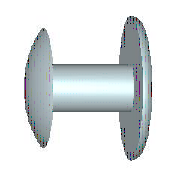
# Autodesk Inventor part: Rivet GB/T 1014-1986-2 X 4
Saved by Autodesk Inventor 2019 (Build 230136000, 136)
## iProperties
IsCustomPart: 0
Company: Autodesk Inc.
Created: 2017-02-09
Part Number: Rivet GB/T 1014-1986-2 X 4
Material: Steel, Mild
Description: Truss head semi - tubuar rivets
Document SubType Name: Modeling
Standard: GB/T 1014-1986
Designer: Autodesk Inc.
Standards Organization: GB
Language: en-US
Size Designation: 2-4
Categories: <MemberInstance><Categories><Category DisplayName="Fasteners" InternalName="e4da775c-781d-43d5-af7c-5136215cf5a6" Mnemonic="FSTN"><Category DisplayName="Rivets" InternalName="cf3d8c00-4198-4f00-854b-0d52b0adb238" Mnemonic="RIVET"><CategoryParameter DisplayName="Nominal Diameter" InternalName="0b221833-a430-4b2f-a4d4-a4e7cdbab5fe" Mnemonic="nomdia"/><CategoryParameter DisplayName="Nominal Length" InternalName="184b63f4-60b5-4ddb-b59d-a876aedee7db" Mnemonic="nomlen"/><CategoryParameter DisplayName="Functional Length" InternalName="2e4ddd0b-69f7-4d63-b45a-ef59153ff940" Mnemonic="fnclen"/><CategoryParameter DisplayName="Type" InternalName="841ce55c-7089-4646-bdbb-4888c77f269c" Mnemonic="type"/><CategoryParameter DisplayName="Grip Range (Min.-Max.)" InternalName="b095e0a4-6026-43f1-9b5f-1a93f7499cb0" Mnemonic="grprng"/></Category></Category><Category DisplayName="DataType" InternalName="23b78d0f-2648-40c6-8793-ca6db495c9e8" Mnemonic="DATATYPE"><CategoryParameter DisplayName="DisplayName" InternalName="05415f3d-3907-474b-a020-eb9d644f4cf3" Mnemonic="DISPLAYNAME"/><CategoryParameter DisplayName="Standard" InternalName="0c0a119c-1e12-4c84-803f-101930972f5e" Mnemonic="STANDARD"/><CategoryParameter DisplayName="Description" InternalName="13903e3d-64b1-4950-80da-f627842ea37f" Mnemonic="DESCRIPTION"/><CategoryParameter DisplayName="Designation" InternalName="2675968c-4ce5-49e0-a4f5-552d29089031" Mnemonic="DESIGNATION"/><CategoryParameter DisplayName="Default Row" InternalName="2af9ec52-faaa-4026-b378-f9fa4afca842" Mnemonic="DEFAULTROW"/><CategoryParameter DisplayName="Folder Name" InternalName="3f06958e-8713-4116-9be7-ed6184ecc97b" Mnemonic="FOLDERNAME"/><CategoryParameter DisplayName="Revision Guid" InternalName="45a75005-10b1-4dfc-8d6d-dfe629f0b93c" Mnemonic="REVISIONGUID"/><CategoryParameter DisplayName="FileName" InternalName="8b46a4cc-9585-4fed-90c3-899f57e09a73" Mnemonic="FILENAME"/><CategoryParameter DisplayName="StdsOrg" InternalName="8f5914e1-4693-403f-8ab5-d37768198c9d" Mnemonic="STDSORG"/><CategoryParameter DisplayName="Family Version" InternalName="914462f6-6e19-4b14-ba84-155b9680b1d0" Mnemonic="FAMILYREVISION"/><CategoryParameter DisplayName="Standard Revision" InternalName="91d5a463-65c2-4fde-b823-3b7fea5e8e17" Mnemonic="STANDARDREVISION"/><CategoryParameter DisplayName="Member Revision" InternalName="a65d44b9-392f-4f4f-857b-e4b3d54996fe" Mnemonic="MEMBERREVISION"/><CategoryParameter DisplayName="ClipFormat" InternalName="bc51e27b-3422-4e78-93ef-cec197ddf230" Mnemonic="CLIPFORMAT"/><CategoryParameter DisplayName="Manufacturer" InternalName="cd6c7a72-a28a-4e50-99a9-2c7f4e13e5ad" Mnemonic="MANUFACTURER"/><CategoryParameter DisplayName="InternalName" InternalName="cf1d0246-76d9-4b4a-8305-fa0409afb5c1" Mnemonic="INTERNALNAME"/><CategoryParameter DisplayName="IsMetric" InternalName="e2385c5b-1ea4-4823-96a8-8de651266ec3" Mnemonic="ISMETRIC"/><Category DisplayName="Part" InternalName="c0e0b642-3bcb-4cc8-9e80-f96d35c4afa4" Mnemonic="PART"><CategoryParameter DisplayName="Part Number" InternalName="016b6077-bfbe-49bd-92c9-d8d59c39c941" Mnemonic="PARTNUMBER"/><CategoryParameter DisplayName="Stock Number" InternalName="4dba7c1c-e26c-444e-836c-b08b433409a8" Mnemonic="STOCKNUMBER"/><CategoryParameter DisplayName="Material Key" InternalName="5c9a8adb-dd2b-4535-b97f-0a94a95fe41f" Mnemonic="MATERIALKEY"/><CategoryParameter DisplayName="Material" InternalName="818a152a-d3c3-49ca-80ee-df7d91421b8e" Mnemonic="MATERIAL"/></Category></Category></Categories><FamilyTemplate Id="Rivet GB_T 1014-1986"><FamilyTemplateParameters><FamilyTemplateParameter ObjectType="kUserParameterObject" ValueType="xs:double" Id="1" ObjectReferenceKey="FLN"/><FamilyTemplateParameter ObjectType="kUserParameterObject" ValueType="xs:double" Id="2" ObjectReferenceKey="INDT"/><FamilyTemplateParameter ObjectType="kUserParameterObject" ValueType="xs:double" Id="3" ObjectReferenceKey="INR"/><FamilyTemplateParameter ObjectType="kUserParameterObject" ValueType="xs:double" Id="4" ObjectReferenceKey="INR2"/><FamilyTemplateParameter ObjectType="kUserParameterObject" ValueType="xs:double" Id="5" ObjectReferenceKey="INT"/><FamilyTemplateParameter ObjectType="kUserParameterObject" ValueType="xs:double" Id="6" ObjectReferenceKey="KOH"/><FamilyTemplateParameter ObjectType="kUserParameterObject" ValueType="xs:double" Id="7" ObjectReferenceKey="NND"/><FamilyTemplateParameter ObjectType="kPartComponentDefinitionObject" ValueType="xs:string" Id="10" SubObjectId="Material"/><FamilyTemplateParameter ObjectType="kPropertyObject" ValueType="xs:string" Id="21" ObjectReferenceKey="{32853F0F-3444-11d1-9E93-0060B03C1CA6}" SubObjectId="5"/><FamilyTemplateParameter ObjectType="kPropertyObject" ValueType="xs:string" Id="22" ObjectReferenceKey="{32853F0F-3444-11d1-9E93-0060B03C1CA6}" SubObjectId="52"/></FamilyTemplateParameters></FamilyTemplate><CategoryParameterMap><ParamToTemplateMap><ParamToTemplate CategoryParameter="//CategoryParameter[@InternalName='cf1d0246-76d9-4b4a-8305-fa0409afb5c1']" ConstantValue="aa952fb0-8e68-4d76-b2e2-4449d269300d"/><ParamToTemplate CategoryParameter="//CategoryParameter[@InternalName='45a75005-10b1-4dfc-8d6d-dfe629f0b93c']" ConstantValue="6c768fb3-c73c-4f69-b849-6390f8207026"/><ParamToTemplate CategoryParameter="//CategoryParameter[@InternalName='3f06958e-8713-4116-9be7-ed6184ecc97b']" ConstantValue="Rivet GB_T 1014-1986"/><ParamToTemplate CategoryParameter="//CategoryParameter[@InternalName='8f5914e1-4693-403f-8ab5-d37768198c9d']" ConstantValue="GB"/><ParamToTemplate CategoryParameter="//CategoryParameter[@InternalName='0c0a119c-1e12-4c84-803f-101930972f5e']" ConstantValue="GB/T 1014-1986"/><ParamToTemplate CategoryParameter="//CategoryParameter[@InternalName='91d5a463-65c2-4fde-b823-3b7fea5e8e17']" TemplateParameter="17"/><ParamToTemplate CategoryParameter="//CategoryParameter[@InternalName='cd6c7a72-a28a-4e50-99a9-2c7f4e13e5ad']" TemplateParameter="18"/><ParamToTemplate CategoryParameter="//CategoryParameter[@InternalName='13903e3d-64b1-4950-80da-f627842ea37f']" ConstantValue="Truss head semi - tubuar rivets"/><ParamToTemplate CategoryParameter="//CategoryParameter[@InternalName='05415f3d-3907-474b-a020-eb9d644f4cf3']" ConstantValue="Rivet GB/T 1014-1986"/><ParamToTemplate CategoryParameter="//CategoryParameter[@InternalName='914462f6-6e19-4b14-ba84-155b9680b1d0']" ConstantValue="11"/><ParamToTemplate CategoryParameter="//CategoryParameter[@InternalName='bc51e27b-3422-4e78-93ef-cec197ddf230']" ConstantValue="CF_INVENTOR.STDPARTS"/><ParamToTemplate CategoryParameter="//CategoryParameter[@InternalName='e2385c5b-1ea4-4823-96a8-8de651266ec3']" ConstantValue="true"/><ParamToTemplate CategoryParameter="//CategoryParameter[@InternalName='2af9ec52-faaa-4026-b378-f9fa4afca842']" ConstantValue="1"/><ParamToTemplate CategoryParameter="//CategoryParameter[@InternalName='8b46a4cc-9585-4fed-90c3-899f57e09a73']" ConstantValue="Rivet GB/T 1014-1986-2 X 4"/><ParamToTemplate CategoryParameter="//CategoryParameter[@InternalName='2675968c-4ce5-49e0-a4f5-552d29089031']" ConstantValue="2 X 4"/><ParamToTemplate CategoryParameter="//CategoryParameter[@InternalName='184b63f4-60b5-4ddb-b59d-a876aedee7db']" TemplateParameter="1"/><ParamToTemplate CategoryParameter="//CategoryParameter[@InternalName='818a152a-d3c3-49ca-80ee-df7d91421b8e']" TemplateParameter="10"/><ParamToTemplate CategoryParameter="//CategoryParameter[@InternalName='0b221833-a430-4b2f-a4d4-a4e7cdbab5fe']" TemplateParameter="7"/><ParamToTemplate CategoryParameter="//CategoryParameter[@InternalName='016b6077-bfbe-49bd-92c9-d8d59c39c941']" TemplateParameter="21"/></ParamToTemplateMap></CategoryParameterMap></MemberInstance>
Mass: 0.288407 g
Surface Area: 1.30796 cm^2
Volume: 0.0367397 cm^3
Density: 7.85 g/cm^3
Appearance: Semi-Polished
Author: Inventor
Autodesk Inventor part; units mm, degrees
ref_plane "YZ Plane" through (0, 0, 0) normal (1, 0, 0) x (0, 1, 0)
ref_plane "XZ Plane" through (0, 0, 0) normal (0, 1, 0) x (-1, 0, 0)
ref_plane "XY Plane" through (0, 0, 0) normal (0, 0, 1) x (1, 0, 0)
sketch "Sketch1" plane through (0, 0, 0) normal (0, 0, 1) x (1, 0, 0)
  line L0 (0, 0) -> (3.0867, 0)
  line L1 (5, 2.988) -> (5, 1)
  line L2 (5, 1) -> (1.1, 1)
  line L3 (1, 1.1) -> (1, 2.49)
  arc A0 (1, 2.49) -> (0, 0) centre (3.6, 0) ccw
  line L4 (0, 0) -> (2.9053, 0)
  arc A1 (1, 1.1) -> (1.1, 1) centre (1.1, 1.1) ccw
  line L5 (5, 2.988) -> (5, 2.988)
  line L6 (5.65, 2.338) -> (5.65, 1.21)
  line L7 (5, 0.56) -> (3.41, 0.56)
  line L8 (3.41, 0.56) -> (3.0867, 0)
  arc A2 (5.65, 2.338) -> (5, 2.988) centre (5, 2.338) ccw
  arc A3 (5, 0.56) -> (5.65, 1.21) centre (5, 1.21) ccw
  point P0 (5.65, 1.4326)
  point P1 (1, 1)
  point P2 (5.65, 2.988)
  point P3 (5.65, 0.56)
  dimension "NND" = 2
  dimension "KOH" = 1
  dimension "FLN" = 4
  dimension "INR" = 0.1
  dimension "INR2" = 3.6
  dimension "KOD" = 4.98
  dimension "d20" = 5.976
  dimension "d21" = 0.65
  dimension "d22" = 60
  dimension "INDT" = 1.12
  dimension "INT" = 2.24
  dimension "d25" = 0.65
  dimension "d26" = 0.65
  constraints: 18 end point, 9 point on line, 8 point on circle, 6 tangent, 4 centre point, 4 perpendicular, 2 parallel, 1 horizontal
  measures "NND" diameter of L2 L4
  measures "KOH" horizontal distance of point (1, 1) L0.start
  measures "FLN" distance of L1.end point (1, 1)
  measures "INR" radius of A1
  measures "INR2" radius of A0
  measures "KOD" diameter of L3.end L4
  measures "d20" diameter of L5 L4
  measures "d21" distance of L1.start point (5.65, 2.988)
  measures "d22" angle of L0 L8
  measures "INDT" diameter of L7 L4
  measures "INT" distance of point (5.65, 0.56) L7.end
  measures "d25" radius of A2
  measures "d26" radius of A3
revolve "Revolution 1" add sketch "Sketch1" angle 360 about axis through (0, 0, 0) along (1, 0, 0)
equation "\"d20\" = 1.2 * KOD"
equation "\"d21\" = 0.65 * KOH"
equation "\"d25\" = 0.65 * KOH"
equation "\"d26\" = 0.65 * KOH"
body "Solid1"
